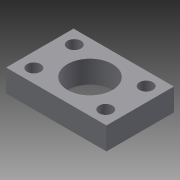
# Autodesk Inventor part: 零件1
Saved by Autodesk Inventor 2014 (Build 180170000, 170)
## iProperties
Created: 2018-10-26
Part Number: 零件1
Material: 常规
Document SubType Name: Modeling
Designer: Administrator
Density: 1 g/cm^3
Appearance: 默认
Author: Administrator
Autodesk Inventor part; units mm, degrees
ref_plane "YZ Plane" through (0, 0, 0) normal (1, 0, 0) x (0, 1, 0)
ref_plane "XZ Plane" through (0, 0, 0) normal (0, 1, 0) x (-1, 0, 0)
ref_plane "XY Plane" through (0, 0, 0) normal (0, 0, 1) x (1, 0, 0)
sketch "草图1" plane through (0, 0, 0) normal (0, 0, 1) x (1, 0, 0)
  line L0 (-33.5, 35.8176) -> (33.5, 35.8176)
  line L1 (33.5, -9.1824) -> (-33.5, -9.1824)
  line L2 (-33.5, -9.1824) -> (-33.5, 35.8176)
  line L3 (33.5, -9.1824) -> (33.5, 35.8176)
  line L4 (0, 46.5629) -> (0, 46.5629)
  line L5 (0, 42.7704) -> (0, -46.1415)
  line L6 (-33.5, 13.3176) -> (96.7396, 13.3176)
  circle A0 centre (-12.4308, 6.5314) radius 0.2107
  circle A1 centre (-24, 26.8176) radius 4.5
  circle A2 centre (-24, -0.1824) radius 4.5
  circle A3 centre (24, -0.1824) radius 4.5
  circle A4 centre (24, 26.8176) radius 4.5
  circle A5 centre (0, 13.3176) radius 15
  point P0 (0, 0)
  dimension "d0" = 67
  dimension "d1" = 45
  dimension "d2" = 27
  dimension "d3" = 48
  dimension "d4" = 9
  dimension "d5" = 30
  constraints: 14 end point, 6 centre point, 3 parallel, 2 perpendicular, 2 point on line, 1 collinear, 1 horizontal, 1 midpoint, 1 symmetric about line, 5 other
  measures "d0" distance of L0.start L0.end
  measures "d1" distance of L1.end L0.start
  measures "d2" distance of A2.centre A1.centre
  measures "d3" distance of A4.centre A1.centre
  measures "d4" diameter of A1
  measures "d5" diameter of A5
extrude "拉伸1" add sketch "草图1" along normal blind 15 contours L0 L5 A5 L6 L2 | L0 L3 L6 A5 L5 | L6 A5 L5 L1 L2 | L3 L1 L5 A5 L6
